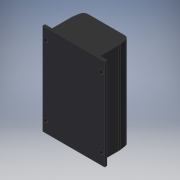
# Autodesk Inventor part: KellyController-KBS-Small
Saved by Autodesk Inventor 2018 (Build 220112000, 112)
## iProperties
Created: 2018-10-11
Part Number: KellyController-KBS-Small
Material: Generic
Document SubType Name: Modeling
Designer: eroldan
Density: 1 g/cm^3
Appearance: Default
Author: eroldan
Autodesk Inventor part; units mm, degrees
ref_plane "YZ Plane" through (0, 0, 0) normal (1, 0, 0) x (0, 1, 0)
ref_plane "XZ Plane" through (0, 0, 0) normal (0, 1, 0) x (-1, 0, 0)
ref_plane "XY Plane" through (0, 0, 0) normal (0, 0, 1) x (1, 0, 0)
sketch "Sketch1" plane through (0, 0, 0) normal (0, 0, 1) x (1, 0, 0)
  line L0 (-38.9, 0) -> (38.9, 0)
  line L1 (-38.9, 0) -> (-38.9, 2.9)
  line L2 (38.9, 0) -> (38.9, 2.9)
  line L3 (-30, 2.9) -> (-38.9, 2.9)
  line L4 (30, 2.9) -> (38.9, 2.9)
  line L5 (30, 2.9) -> (30, 27.9)
  line L6 (-30, 2.9) -> (-30, 27.9)
  line L7 (-30, 27.9) -> (30, 27.9) construction
  line L8 (-28, 41) -> (28, 41)
  line L9 (-30, 27.9) -> (-28, 41)
  line L10 (30, 27.9) -> (28, 41)
  point P0 (0, 0)
  point P1 (0, 0)
  point P2 (0, 27.9)
  point P3 (0, 41)
  dimension "d0" = 77.8
  dimension "d1" = 2.9
  dimension "d6" = 25
  dimension "d7" = 56
  dimension "d8" = 41
  constraints: 22 end point, 4 vertical, 3 midpoint, 3 perpendicular, 2 horizontal, 2 vertical alignment, 1 coincident
  measures "d0" distance of L0.start L0.end
  measures "d1" distance of L0.start L1.end
  measures "d6" distance of L4.start L5.end
  measures "d7" distance of L8.start L8.end
  measures "d8" distance between parallel lines of L0 L8
extrude "Extrusion1" add sketch "Sketch1" along normal blind 115
fillet "Fillet1" radius 5.75 2 edges at (28, 41, 57.5) (-28, 41, 57.5)
fillet "Fillet2" radius 20 2 edges at (-30, 27.9, 57.5) (30, 27.9, 57.5)
sketch "Sketch2" plane through (-38.9, 0, 0) normal (0, -1, 0) x (1, 0, 0)
  line L0 (0, 0) -> (77.8, 0) projected
  line L1 (0, 0) -> (0, 115) projected
  line L2 (77.8, 0) -> (77.8, 115) projected
  line L3 (0, 115) -> (77.8, 115) projected
  point P0 (38.9, 0)
  point P1 (4, 13.75)
  point P2 (73.8, 13.75)
  point P3 (4, 101)
  point P4 (73.8, 101)
  dimension "d11" = 13.75
  dimension "d12" = 4
  dimension "d13" = 4
  dimension "d14" = 14
  measures "d11" distance from line of L0 point (4, 13.75)
  measures "d12" distance from line of L1 point (4, 13.75)
  measures "d13" distance from line of L2 point (73.8, 13.75)
  measures "d14" distance from line of L3 point (4, 101)
hole "Hole1" at (-34.9, 0, 13.75) at (34.9, 0, 13.75) at (-34.9, 0, 101) at (34.9, 0, 101) direction (0, 1, 0) diameter 4.7 end through all
sketch "Sketch3" plane through (0, 0, 0) normal (0, 0, -1) x (-1, 0, 0)
  circle A0 centre (20.3461, 28.3) radius 2.425
  circle A1 centre (20.3461, 22.3) radius 2.425
  line L0 (-23.0612, 41) -> (23.0612, 41) projected
  point P0 (0, 0)
  dimension "d22" = 4.85
  dimension "d23" = 4.85
  dimension "d24" = 6
  dimension "d25" = 12.7
  constraints: 2 centre point, 1 vertical alignment
  measures "d22" diameter of A0
  measures "d23" diameter of A1
  measures "d24" distance of A1.centre A0.centre
  measures "d25" distance from line of L0 A0.centre
extrude "Extrusion2" add sketch "Sketch3" along normal blind 6.5
fillet "Fillet3" radius 2.25 2 edges at (-17.9211, 28.3, -6.5) (-17.9211, 22.3, -6.5)
equation "\"d13\" = d12"
equation "\"d23\" = d22"
body "Solid1"
